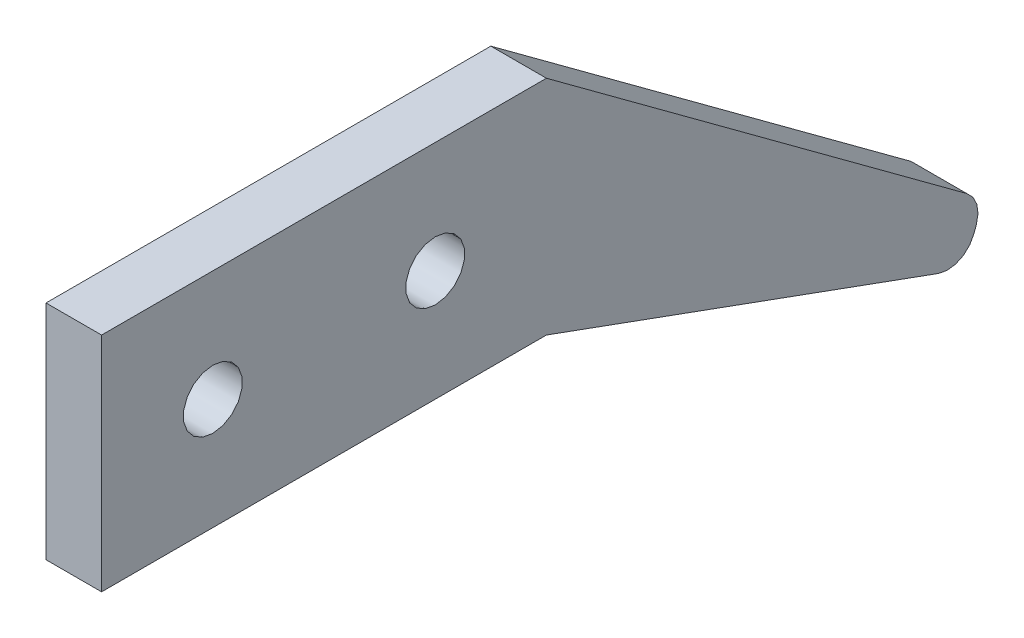
# Autodesk Inventor part: ramp gusset
Saved by Autodesk Inventor 2016 (Build 200138000, 138)
## iProperties
Created: 2016-02-06
Part Number: ramp gusset
Material: Aluminum 6061
Document SubType Name: Modeling
Designer: gus
Density: 2.7 g/cm^3
Appearance: Aluminum - Flat
Author: gus
Autodesk Inventor part; units mm, degrees
ref_plane "YZ Plane" through (0, 0, 0) normal (1, 0, 0) x (0, 1, 0)
ref_plane "XZ Plane" through (0, 0, 0) normal (0, 1, 0) x (-1, 0, 0)
ref_plane "XY Plane" through (0, 0, 0) normal (0, 0, 1) x (1, 0, 0)
sketch "Sketch1" plane through (0, 0, 0) normal (1, 0, 0) x (0, 1, 0)
  line L0 (0, 0) -> (0, -50.8)
  line L1 (0, -50.8) -> (-36.8076, -100.7082)
  line L2 (-42.7746, -98.5364) -> (-25.4, -50.8)
  line L3 (-25.4, -50.8) -> (-25.4, 0)
  line L4 (0, 0) -> (-25.4, 0)
  line L5 (-42.7746, -98.5364) -> (-36.8076, -100.7082)
  circle A0 centre (-12.7, -38.1) radius 3.3734
  circle A1 centre (-12.7, -12.7) radius 3.3734
  dimension "d0" = 50.8
  dimension "d4" = 160
  dimension "d5" = 50.8
  dimension "d6" = 6.35
  dimension "d7" = 25.4
  dimension "d8" = 6.7469
  dimension "d9" = 6.7469
  dimension "d10" = 12.7
  dimension "d11" = 38.1
  dimension "d12" = 12.7
  dimension "d13" = 12.7
  constraints: 12 end point, 2 centre point, 2 vertical, 1 horizontal, 1 parallel, 1 perpendicular
  measures "d0" distance of L0.start L0.end
  measures "d4" angle of L2 L3
  measures "d5" distance of L2.start L2.end
  measures "d6" distance of L2.start L1.end
  measures "d7" distance of L0.start L3.end
  measures "d8" diameter of A0
  measures "d9" diameter of A1
  measures "d10" distance from line of L3 A0.centre
  measures "d11" distance from line of L4 A0.centre
  measures "d12" distance from line of L4 A1.centre
  measures "d13" distance from line of L3 A1.centre
extrude "Extrusion1" add sketch "Sketch1" along normal blind 6.35
fillet "Fillet1" radius 3.175 2 edges at (3.175, -42.7746, -98.5364) (3.175, -36.8076, -100.7082)
body "Solid1"
